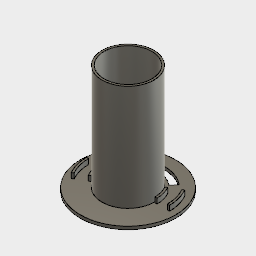
Gelatin_Mold_Top v2 (Autodesk Fusion 360 design; units mm, degrees)
Autodesk Fusion 360 part; units mm, degrees
sketch "Sketch1" plane through (0, 0, 0) normal (0, 1, 0) x (1, 0, 0)
  circle A0 centre (0, 0) radius 46
  dimension "d1" = 92
  measures "d1" diameter of A0
extrude "Extrude1" add sketch "Sketch1" along normal blind 3
sketch "Sketch2" plane through (0, 3, 0) normal (0, 1, 0) x (-1, 0, 0)
  circle A0 centre (0, 0) radius 46
  arc A1 (40, 0.0207) -> (34.641, 20) centre (0, 0) ccw
  arc A2 (-40, 0.0207) -> (-34.641, -20) centre (0, 0) ccw
  arc A3 (38, 0.0207) -> (32.909, 19) centre (0, 0) ccw
  arc A4 (-38, 0.0207) -> (-32.909, -19) centre (0, 0) ccw
  arc A5 (28, 0.0207) -> (24.2487, 14) centre (0, 0) ccw
  arc A6 (-28, 0.0207) -> (-24.2487, -14) centre (0, 0) ccw
  arc A7 (26, 0.0207) -> (22.5167, 13) centre (0, 0) ccw
  arc A8 (-26, 0.0207) -> (-22.5167, -13) centre (0, 0) ccw
  line L0 (-22.5167, -13) -> (-24.2487, -14)
  line L1 (-32.909, -19) -> (-34.641, -20)
  line L2 (-26, 0.0207) -> (-28, 0.0207)
  line L3 (-38, 0.0207) -> (-40, 0.0207)
  line L4 (0.0359, 0.0207) -> (0, 0)
  line L5 (40, 0.0207) -> (38, 0.0207)
  line L6 (28, 0.0207) -> (26, 0.0207)
  line L7 (34.641, 20) -> (32.909, 19)
  line L8 (24.2487, 14) -> (22.5167, 13)
  dimension "d8" = 30
  dimension "d9" = 30
  measures "d8" angle of L0 L5
  measures "d9" angle of L5 L7
extrude "Extrude2" add sketch "Sketch2" along normal blind 5 contours A1 A3 L5 L7 | A2 A4 L1 L3 | A5 A7 L6 L8 | A6 A8 L0 L2
sketch "Sketch3" plane through (0, 3, 0) normal (0, 1, 0) x (-1, 0, 0)
  line L0 (40, 0.0207) -> (38, 0.0207)
  arc A0 (38, 0.0207) -> (32.909, 19) centre (0, 0) ccw
  line L1 (32.909, 19) -> (34.641, 20)
  arc A1 (40, 0.0207) -> (34.641, 20) centre (0, 0) ccw
  line L2 (-32.909, -19) -> (-34.641, -20)
  arc A2 (-40, 0.0207) -> (-34.641, -20) centre (0, 0) ccw
  line L3 (-40, 0.0207) -> (-38, 0.0207)
  arc A3 (-38, 0.0207) -> (-32.909, -19) centre (0, 0) ccw
  line L4 (28, 0.0207) -> (26, 0.0207)
  arc A4 (26, 0.0207) -> (22.5167, 13) centre (0, 0) ccw
  line L5 (22.5167, 13) -> (24.2487, 14)
  arc A5 (28, 0.0207) -> (24.2487, 14) centre (0, 0) ccw
  line L6 (-22.5167, -13) -> (-24.2487, -14)
  arc A6 (-28, 0.0207) -> (-24.2487, -14) centre (0, 0) ccw
  line L7 (-28, 0.0207) -> (-26, 0.0207)
  arc A7 (-26, 0.0207) -> (-22.5167, -13) centre (0, 0) ccw
  circle A8 centre (0, 0) radius 46
  line L8 (-17.9147, -21.5189) -> (-22.3933, -26.8987)
  line L9 (21.6604, -17.7433) -> (27.1948, -22.0328)
  arc A9 (-22.3933, -26.8987) -> (27.1948, -22.0328) centre (0, 0) ccw
  arc A10 (-17.9147, -21.5189) -> (21.6604, -17.7433) centre (0, 0) ccw
  arc A11 (28, 0.0207) -> (24.2487, 14) centre (0, 0) ccw
  arc A12 (-28, 0.0207) -> (-24.2487, -14) centre (0, 0) ccw
  dimension "d14" = 92
  measures "d14" angle of L8 L9
extrude "Extrude3" cut sketch "Sketch3" against normal blind 3 contours L8 L9 A9 A10
sketch "Sketch4" plane through (0, 3, 0) normal (0, 1, 0) x (-1, 0, 0)
  line L0 (21.6604, -17.7433) -> (27.1948, -22.0328)
  arc A0 (-22.3933, -26.8987) -> (27.1948, -22.0328) centre (0, 0) ccw
  line L1 (-22.3933, -26.8987) -> (-17.9147, -21.5189)
  arc A1 (-17.9147, -21.5189) -> (21.6604, -17.7433) centre (0, 0) ccw
  line L2 (40, 0.0207) -> (38, 0.0207)
  arc A2 (38, 0.0207) -> (32.909, 19) centre (0, 0) ccw
  line L3 (32.909, 19) -> (34.641, 20)
  arc A3 (40, 0.0207) -> (34.641, 20) centre (0, 0) ccw
  line L4 (-32.909, -19) -> (-34.641, -20)
  arc A4 (-40, 0.0207) -> (-34.641, -20) centre (0, 0) ccw
  line L5 (-40, 0.0207) -> (-38, 0.0207)
  arc A5 (-38, 0.0207) -> (-32.909, -19) centre (0, 0) ccw
  line L6 (28, 0.0207) -> (26, 0.0207)
  arc A6 (26, 0.0207) -> (22.5167, 13) centre (0, 0) ccw
  line L7 (22.5167, 13) -> (24.2487, 14)
  arc A7 (28, 0.0207) -> (24.2487, 14) centre (0, 0) ccw
  line L8 (-22.5167, -13) -> (-24.2487, -14)
  arc A8 (-28, 0.0207) -> (-24.2487, -14) centre (0, 0) ccw
  line L9 (-28, 0.0207) -> (-26, 0.0207)
  arc A9 (-26, 0.0207) -> (-22.5167, -13) centre (0, 0) ccw
  circle A10 centre (0, 0) radius 46
  circle A11 centre (0, 0) radius 25
  circle A12 centre (0, 0) radius 23
  dimension "d17" = 50
  dimension "d18" = 46
  measures "d17" diameter of A11
  measures "d18" diameter of A12
extrude "Extrude4" add sketch "Sketch4" along normal blind 102 contours A11
